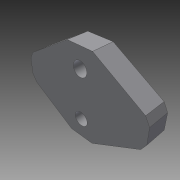
# Autodesk Inventor part: z_axis_top_cap
Saved by Autodesk Inventor 2014 (Build 180170000, 170)
## iProperties
Created: 2014-04-16
Part Number: z_axis_top_cap
Material: Plywood, Finish
Document SubType Name: Modeling
Designer: buben
Density: 0.552 g/cm^3
Appearance: Plywood - New
Author: buben
Autodesk Inventor part; units mm, degrees
ref_plane "YZ Plane" through (0, 0, 0) normal (1, 0, 0) x (0, 1, 0)
ref_plane "XZ Plane" through (0, 0, 0) normal (0, 1, 0) x (-1, 0, 0)
ref_plane "XY Plane" through (0, 0, 0) normal (0, 0, 1) x (1, 0, 0)
sketch "Sketch1" plane through (0, 0, 0) normal (0, 1, 0) x (-1, 0, 0)
  line L0 (4, -13.5) -> (-4, -13.5)
  line L1 (-4, -13.5) -> (-20, -4)
  line L2 (-20, -4) -> (-20, 4)
  line L3 (-20, 4) -> (-4, 13.5)
  line L4 (-4, 13.5) -> (4, 13.5)
  line L5 (4, 13.5) -> (20, 4)
  line L6 (20, 4) -> (20, -4)
  line L7 (20, -4) -> (4, -13.5)
  circle A0 centre (0, -7.5) radius 2.25
  circle A1 centre (0, 7.5) radius 2.25
  circle A2 centre (0, -7.5) radius 4.5 construction
  circle A3 centre (0, 7.5) radius 4.5 construction
  circle A4 centre (11.5, 0) radius 4 construction
  circle A5 centre (-11.5, 0) radius 4 construction
  point P0 (0, 0)
  point P1 (0, -13.5)
  point P2 (0, 13.5)
  point P3 (20, 0)
  point P4 (-20, 0)
  dimension "d1" = 4.5
  dimension "d2" = 15
  dimension "d3" = 7.5
  dimension "d4" = 9
  dimension "d5" = 8
  dimension "d6" = 23
  dimension "d7" = 11.5
  dimension "d8" = 20
  dimension "d9" = 20
  dimension "d10" = 6
  dimension "d11" = 8
  dimension "d12" = 8
  constraints: 16 end point, 6 centre point, 4 horizontal alignment, 4 midpoint, 4 vertical alignment, 3 equal length, 3 equal radius, 2 coincident, 2 parallel, 1 horizontal, 1 perpendicular
  measures "d1" diameter of A0
  measures "d2" distance of A1.centre A0.centre
  measures "d3" distance of point (0, 0) A0.centre
  measures "d4" diameter of A2
  measures "d5" diameter of A4
  measures "d6" distance of A5.centre A4.centre
  measures "d7" distance of point (0, 0) A4.centre
  measures "d8" distance from line of L6 point (0, 0)
  measures "d9" distance from line of L2 point (0, 0)
  measures "d10" distance from line of L4 A1.centre
  measures "d11" distance of L3.end L4.end
  measures "d12" distance of L5.end L6.end
extrude "Extrusion1" add sketch "Sketch1" along normal blind 6.5
chamfer "Chamfer1" distance 1.5 angle 45 4 edges at (20, 3.25, 4) (20, 3.25, -4) (-20, 3.25, -4) (-20, 3.25, 4)
equation "\"d3\" = 0.5 * d2"
equation "\"d7\" = 0.5 * d6"
equation "\"d9\" = d8"
body "Solid1"
